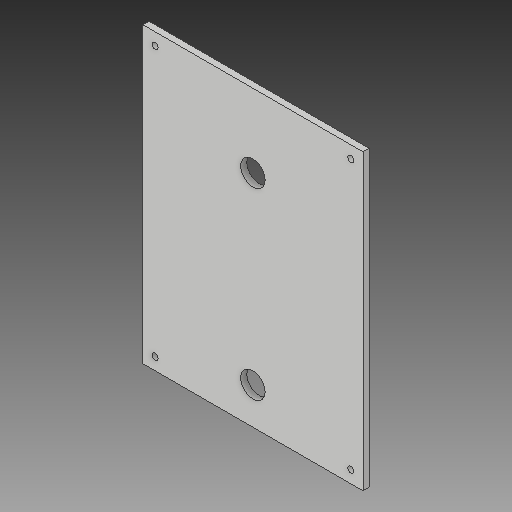
# Autodesk Inventor part: GearBoxRearPlate
Saved by Autodesk Inventor 2019 (Build 230136000, 136)
## iProperties
Created: 2018-10-28
Part Number: GearBoxRearPlate
Material: Generic
Document SubType Name: Modeling
Designer: Swapnil
Density: 1 g/cm^3
Appearance: Default
Mass: 54.4014 g
Surface Area: 363.422 cm^2
Volume: 54.4014 cm^3
Author: Swapnil
Autodesk Inventor part; units mm, degrees
ref_plane "YZ Plane" through (0, 0, 0) normal (1, 0, 0) x (0, 1, 0)
ref_plane "XZ Plane" through (0, 0, 0) normal (0, 1, 0) x (-1, 0, 0)
ref_plane "XY Plane" through (0, 0, 0) normal (0, 0, 1) x (1, 0, 0)
sketch "Sketch1" plane through (0, 0, 0) normal (0, 0, 1) x (1, 0, 0)
  line L0 (0, 0) -> (0, 40.5449) construction
  line L1 (0, 0) -> (42.3786, 0) construction
  line L2 (-57.15, 76.2) -> (57.15, 76.2)
  line L3 (57.15, 76.2) -> (57.15, -76.2)
  line L4 (57.15, -76.2) -> (-57.15, -76.2)
  line L5 (-57.15, -76.2) -> (-57.15, 76.2)
  dimension "d0" = 152.4
  dimension "d1" = 114.3
  constraints: 12 end point, 2 horizontal, 2 parallel, 1 perpendicular, 1 vertical, 2 other
  measures "d0" distance of L2.end L3.end
  measures "d1" distance of L2.start L2.end
extrude "Extrusion1" add sketch "Sketch1" along normal blind 3.175
sketch "Sketch2" plane through (0, 0, 3.175) normal (0, 0, 1) x (1, 0, 0)
  line L0 (57.15, 76.2) -> (-57.15, 76.2) projected
  line L1 (-57.15, 76.2) -> (-57.15, -76.2) projected
  point P0 (0, 0)
  point P1 (0, 38.1)
  dimension "d4" = 38.1
  dimension "d5" = 57.15
  measures "d4" distance from line of L0 point (0, 38.1)
  measures "d5" distance from line of L1 point (0, 38.1)
hole "Hole1" at (0, 38.1, 3.175) direction (0, 0, -1) diameter 12.7 end through all
sketch "Sketch3" plane through (0, 0, 3.175) normal (0, 0, 1) x (1, 0, 0)
  line L0 (-57.15, -76.2) -> (57.15, -76.2) projected
  line L1 (-57.15, 76.2) -> (-57.15, -76.2) projected
  point P0 (0, 0)
  point P1 (-50.8, -69.85)
  dimension "d13" = 6.35
  dimension "d14" = 6.35
  measures "d13" distance from line of L0 point (-50.8, -69.85)
  measures "d14" distance from line of L1 point (-50.8, -69.85)
hole "Hole2" at (-50.8, -69.85, 3.175) direction (0, 0, -1) diameter 3.175 end through all
mirror "Mirror1" about plane through (0, 0, 0) normal (1, 0, 0) of "Hole2"
mirror "Mirror2" about plane through (0, 0, 0) normal (0, 1, 0) of "Hole2", "Mirror1"
sketch "Sketch4" plane through (0, 0, 3.175) normal (0, 0, 1) x (1, 0, 0)
  line L0 (-57.15, -76.2) -> (57.15, -76.2) projected
  line L1 (-57.15, 76.2) -> (-57.15, -76.2) projected
  point P0 (0, 0)
  point P1 (0, -57.15)
  dimension "d22" = 19.05
  dimension "d23" = 57.15
  measures "d22" distance from line of L0 point (0, -57.15)
  measures "d23" distance from line of L1 point (0, -57.15)
hole "Hole3" at (0, -57.15, 3.175) direction (0, 0, -1) diameter 12.7 end through all
body "Solid1"
